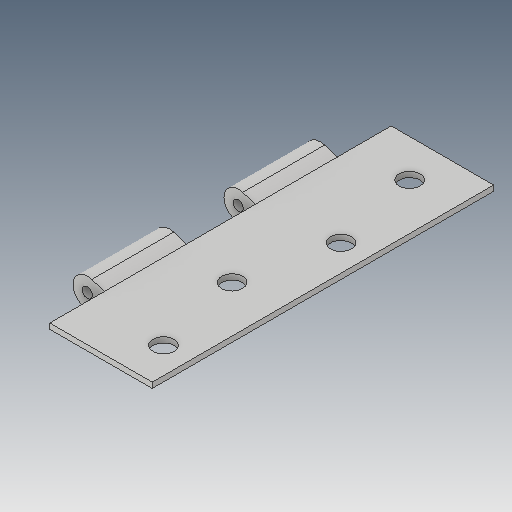
# Autodesk Inventor part: 蝶番1
Saved by Autodesk Inventor 2020.3 (Build 243373000, 373)
## iProperties
Part Number: 蝶番1
Material: 一般
Document SubType Name: Modeling
Designer: highs
Density: 1 g/cm^3
Appearance: 既定
Author: highs
Autodesk Inventor part; units mm, degrees
ref_plane "YZ Plane" through (0, 0, 0) normal (1, 0, 0) x (0, 1, 0)
ref_plane "XZ Plane" through (0, 0, 0) normal (0, 1, 0) x (-1, 0, 0)
ref_plane "XY Plane" through (0, 0, 0) normal (0, 0, 1) x (1, 0, 0)
sketch "スケッチ1" plane through (0, 0, 0) normal (0, 0, 1) x (1, 0, 0)
  line L0 (0, 0) -> (30, 0)
  line L1 (30, 0) -> (30, -1.6)
  line L2 (30, -1.6) -> (0, -1.6)
  arc A0 (-3.7104, 1.1971) -> (-1.0982, -1.2457) centre (-5, -2.8) ccw
  line L3 (0, 0) -> (-3.7104, 1.1971)
  line L4 (0, -1.6) -> (-1.0982, -1.2457)
  line L5 (0, 0) -> (0, -1.6) construction
  circle A1 centre (-5, -2.8) radius 1.5
  dimension "d0" = 1.6
  dimension "d1" = 30
  dimension "d2" = 8.4
  dimension "d4" = 35
  dimension "d5" = 2.8
  dimension "d6" = 3
  constraints: 12 end point, 2 centre point, 2 perpendicular, 2 point on circle, 1 coincident, 1 horizontal, 1 parallel, 1 tangent, 1 vertical
  measures "d0" distance between parallel lines of L2 L0
  measures "d1" distance of L0.start L0.end
  measures "d2" diameter of A0
  measures "d4" distance from line of L1 A0.centre
  measures "d5" distance from line of A0.centre L0
  measures "d6" diameter of A1
extrude "押し出し1" add sketch "スケッチ1" along normal blind 100
sketch "スケッチ2" plane through (0, -1.6, 0) normal (0, -1, 0) x (1, 0, 0)
  line L0 (0, 100) -> (-3.7104, 100) projected
  line L1 (0, 100) -> (-10, 100)
  line L2 (-10, -0.2) -> (0, -0.2)
  line L3 (-10, 84) -> (0, 84)
  line L4 (0, 0) -> (0, 100) projected
  line L5 (-10, 39.8) -> (0, 39.8)
  line L6 (-10, 15.8) -> (0, 15.8)
  line L7 (16.4, 101.8084) -> (16.4, 1.6084) construction
  line L8 (30, 0) -> (30, 100) construction
  line L9 (30, 89) -> (16.4, 89) construction
  line L10 (30, 63) -> (16.4, 63) construction
  line L11 (30, 37) -> (16.4, 37) construction
  line L12 (30, 11) -> (16.4, 11) construction
  line L13 (30, 100) -> (0, 100) construction
  line L14 (22.3, 100) -> (22.3, 0) construction
  circle A0 centre (22.3, 89) radius 3.1
  circle A1 centre (16.4, 63) radius 3.1
  circle A2 centre (22.3, 37) radius 3.1
  circle A3 centre (16.4, 11) radius 3.1
  line L15 (30, 0) -> (0, 0) construction
  line L16 (-10, 60) -> (0, 60)
  line L17 (-10, 100) -> (-10, 84)
  line L18 (0, 84) -> (0, 100)
  line L19 (-10, 60) -> (-10, 39.8)
  line L20 (-10, 15.8) -> (-10, -0.2)
  line L21 (0, -0.2) -> (0, 15.8)
  line L22 (0, 39.8) -> (0, 60)
  dimension "d9" = 100.2
  dimension "d10" = 10
  dimension "d11" = 16
  dimension "d12" = 16
  dimension "d13" = 24
  dimension "d15" = 7.7
  dimension "d16" = 6.2
  dimension "d17" = 11
  dimension "d19" = 11
  dimension "d20" = 13.6
  dimension "d21" = 37
  dimension "d22" = 37
  dimension "d23" = 24
  constraints: 36 end point, 15 perpendicular, 14 point on line, 11 parallel, 4 centre point, 3 collinear, 3 equal radius, 2 coincident, 2 horizontal, 2 vertical
  measures "d9" distance of L1.end L2.start
  measures "d10" distance of L2.start L2.end
  measures "d11" distance between parallel lines of L3 L1
  measures "d12" distance between parallel lines of L2 L6
  measures "d13" distance between parallel lines of L6 L5
  measures "d15" distance between parallel lines of L8 L14
  measures "d16" diameter of A0
  measures "d17" distance between parallel lines of L13 L9
  measures "d19" distance between parallel lines of L15 L12
  measures "d20" distance between parallel lines of L8 L7
  measures "d21" distance from line of L15 A2.centre
  measures "d22" distance from line of L13 A1.centre
  measures "d23" distance between parallel lines of L16 L3
extrude "押し出し2" cut sketch "スケッチ2" along normal mid plane 100.2
